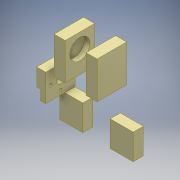
# Autodesk Inventor part: Cuerpo
Saved by Autodesk Inventor 2016 (Build 200138000, 138)
## iProperties
Created: 2019-03-15
Part Number: Cuerpo
Material: Nilón 6/6
Document SubType Name: Modeling
Designer: FIMCP
Mass: 57.9207 g
Surface Area: 176.212 cm^2
Volume: 51.2572 cm^3
Density: 1.13 g/cm^3
Appearance: Nilón 6
Author: FIMCP
Autodesk Inventor part; units mm, degrees
ref_plane "YZ Plane" through (0, 0, 0) normal (1, 0, 0) x (0, 1, 0)
ref_plane "XZ Plane" through (0, 0, 0) normal (0, 1, 0) x (-1, 0, 0)
ref_plane "XY Plane" through (0, 0, 0) normal (0, 0, 1) x (1, 0, 0)
sketch "Boceto2" plane through (0, 0, 0) normal (0, 1, 0) x (-1, 0, 0)
  line L0 (20, 72.2842) -> (13, 72.2842)
  line L1 (20, 72.2842) -> (13, 72.2842) projected
  line L2 (13, 72.2842) -> (20, 72.2842)
  line L3 (25, 27.0002) -> (13.1036, 27.0002)
  line L4 (13.1036, 27.0002) -> (13, 72.2842)
  line L5 (-8, 72.2842) -> (-20, 72.2842)
  line L6 (-23, 27.0002) -> (-8, 27.0002)
  line L7 (-8, 27.0002) -> (-8, 72.2842)
  line L8 (13.1036, 27.0002) -> (25, 27.0002)
  line L9 (25, 27.0002) -> (25, 70.7107)
  line L10 (20, 72.2842) -> (13.1036, 72.2842)
  line L11 (-8, 27.0002) -> (-23, 27.0002)
  line L12 (-23, 27.0002) -> (-23, 71.3863)
  line L13 (-20, 72.2842) -> (-8, 72.2842)
  line L14 (-8, 72.2842) -> (-8, 27.0002)
  arc A0 (-20, 72.2842) -> (-23, 71.3863) centre (0, 0) ccw
  arc A1 (25, 70.7107) -> (20, 72.2842) centre (0, 0) ccw
  constraints: 28 end point, 5 horizontal, 5 parallel, 5 point on circle, 2 centre point, 2 perpendicular, 1 coincident, 1 point on line
extrude "Extrusión2" add sketch "Boceto2" against normal blind 32 contours A1 L9 L3 L4 L0
sketch "Boceto3" plane through (0, 0, 0) normal (0, 1, 0) x (-1, 0, 0)
  line L0 (-40, 8) -> (-40, -42) projected
  line L1 (-40, -3) -> (-15, -3)
  line L2 (-15, -3) -> (-15, -31)
  line L3 (-15, -31) -> (-40, -31)
  line L4 (-40, -31) -> (-40, -3)
  line L5 (39.9026, -3) -> (14.9026, -3)
  line L6 (14.9026, -3) -> (14.9026, -31)
  line L7 (14.9026, -31) -> (39.9026, -31)
  line L8 (39.9026, -31) -> (39.9026, -3)
  line L9 (-40, 8) -> (-55, 8) projected
  line L10 (55, 8) -> (40, 8) projected
  point P0 (0, 0)
  dimension "d27" = 25
  dimension "d28" = 28
  dimension "d30" = 25
  dimension "d31" = 28
  dimension "d65" = 11
  dimension "d66" = 11
  constraints: 16 end point, 4 parallel, 2 horizontal, 2 perpendicular, 1 point on line
  measures "d27" distance of L2.end L3.end
  measures "d28" distance of L1.end L2.end
  measures "d30" distance of L7.end L6.end
  measures "d31" distance of L6.end L5.end
  measures "d65" distance between parallel lines of L9 L1
  measures "d66" distance between parallel lines of L10 L5
extrude "Extrusión3" add sketch "Boceto3" against normal blind 11
sketch "Boceto4" plane through (0, 0, 0) normal (0, 1, 0) x (-1, 0, 0)
  line L0 (34.104, 26.8434) -> (43.9649, 26.8434)
  line L1 (43.9649, 26.8434) -> (43.9649, 8)
  line L2 (40, -2.8934) -> (34.1721, -2.8934)
  line L3 (34.1721, -2.8934) -> (34.104, 26.8434)
  line L4 (13.1036, 27.0002) -> (13, 72.2842) projected
  line L5 (55, 8) -> (40, 8) projected
  line L6 (40, 8) -> (40, -42) projected
  line L7 (43.9649, 8) -> (40, 8)
  line L8 (40, 8) -> (40, -2.8934)
  line L9 (43.9649, 5.0585) -> (44, 5.0585)
  point P0 (0, 0)
  dimension "d37" = 21
  constraints: 14 end point, 3 point on line, 2 horizontal, 2 parallel, 2 perpendicular, 1 other
  measures "d37" distance between parallel lines of L4 L3
extrude "Extrusión4" add sketch "Boceto4" against normal blind 32
sketch "Boceto5" plane through (0, 0, 0) normal (1, 0, 0) x (0, 1, 0)
  circle A0 centre (-16, 51.2842) radius 11
  line L0 (0, 72.2842) -> (-32, 72.2842) projected
  line L1 (2, -75) -> (2, 72.808) projected
  point P0 (0, 0)
  point P1 (2, 72.2842)
  dimension "d40" = 22
  dimension "d41" = 21
  dimension "d42" = 18
  constraints: 1 centre point
  measures "d40" diameter of A0
  measures "d41" distance from line of L0 A0.centre
  measures "d42" distance from line of L1 A0.centre
extrude "Extrusión5" cut sketch "Boceto5" along normal mid plane 38
sketch "Boceto8" plane through (0, 0, 0) normal (0, 1, 0) x (-1, 0, 0)
  line L0 (59.5508, 67.2842) -> (-59.748, 67.2842)
  line L1 (-59.748, 67.2842) -> (-59.748, 82.2842)
  line L2 (-59.748, 82.2842) -> (59.5508, 82.2842)
  line L3 (59.5508, 82.2842) -> (59.5508, 67.2842)
  line L4 (13, 72.2842) -> (20, 72.2842) projected
  point P0 (0, 0)
  dimension "d67" = 15
  dimension "d71" = 5
  constraints: 8 end point, 2 parallel, 1 horizontal, 1 perpendicular
  measures "d67" distance of L0.end L1.end
  measures "d71" distance between parallel lines of L4 L0
extrude "Extrusión8" cut sketch "Boceto8" along normal mid plane 70
sketch "Boceto12" plane through (0, 0, 0) normal (1, 0, 0) x (0, 1, 0)
  circle A0 centre (-16, 12.1066) radius 4
  line L0 (0, 54.8927) -> (0, 4.9968) projected
  line L1 (0, -2.8934) -> (-32, -2.8934) projected
  circle A1 centre (-5, 12.0585) radius 1.5
  line L2 (-32, 67.2842) -> (-32, -75) projected
  circle A2 centre (-27, 12.1066) radius 1.5
  circle A3 centre (-16, 2.1066) radius 1.5
  circle A4 centre (-16, 20.6066) radius 1.5
  point P0 (0, 0)
  point P1 (0, -2.9415)
  dimension "d95" = 8
  dimension "d96" = 16
  dimension "d97" = 15
  dimension "d98" = 3
  dimension "d99" = 5
  dimension "d102" = 3
  dimension "d103" = 5
  dimension "d104" = 3
  dimension "d105" = 5
  dimension "d106" = 3
  dimension "d107" = 16
  dimension "d108" = 16
  dimension "d109" = 15
  dimension "d110" = 23.5
  constraints: 5 centre point, 1 other
  measures "d95" diameter of A0
  measures "d96" distance from line of A0.centre L0
  measures "d98" diameter of A1
  measures "d99" distance from line of L0 A1.centre
  measures "d102" diameter of A2
  measures "d103" distance from line of L2 A2.centre
  measures "d104" diameter of A3
  measures "d106" diameter of A4
  measures "d107" distance from line of L0 A3.centre
  measures "d108" distance from line of L0 A4.centre
extrude "Extrusión12" cut sketch "Boceto12" against normal blind 50
sketch "Boceto15" plane through (0, 0, 0) normal (0, 1, 0) x (-1, 0, 0)
  line L0 (-21.8152, 26.9203) -> (-9.8152, 26.9203)
  line L1 (-9.8152, 26.9203) -> (-9.8152, 67.2842)
  line L2 (-9.8152, 67.2842) -> (-21.8152, 67.2842)
  line L3 (-21.8152, 67.2842) -> (-21.8152, 26.9203)
  point P0 (0, 0)
  dimension "d128" = 12
  constraints: 8 end point, 2 parallel, 1 horizontal, 1 perpendicular
  measures "d128" distance of L2.end L1.end
extrude "Extrusión15" add sketch "Boceto15" against normal blind 32
